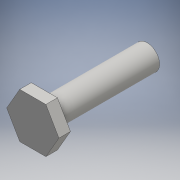
# Autodesk Inventor part: bolt
Saved by Autodesk Inventor 2016 (Build 200138000, 138)
## iProperties
Created: 2017-05-26
Part Number: bolt
Material: Ogólny
Document SubType Name: Modeling
Designer: Karol
Density: 1 g/cm^3
Appearance: Domyślna
Author: Karol
Autodesk Inventor part; units mm, degrees
ref_plane "YZ Plane" through (0, 0, 0) normal (1, 0, 0) x (0, 1, 0)
ref_plane "XZ Plane" through (0, 0, 0) normal (0, 1, 0) x (-1, 0, 0)
ref_plane "XY Plane" through (0, 0, 0) normal (0, 0, 1) x (1, 0, 0)
sketch "Sketch1" plane through (0, 0, 0) normal (0, 1, 0) x (-1, 0, 0)
  circle A0 centre (0, 0) radius 1.5
  dimension "d0" = 3
  constraints: 1 centre point, 1 coincident
  measures "d0" diameter of A0
extrude "Extrusion1" add sketch "Sketch1" along normal blind 12.5
sketch "Sketch2" plane through (0, 0, 0) normal (0, -1, 0) x (1, 0, 0)
  line L0 (3.1754, 0) -> (1.5877, -2.75)
  line L1 (1.5877, -2.75) -> (-1.5877, -2.75)
  line L2 (-1.5877, -2.75) -> (-3.1754, 0)
  line L3 (-3.1754, 0) -> (-1.5877, 2.75)
  line L4 (-1.5877, 2.75) -> (1.5877, 2.75)
  line L5 (1.5877, 2.75) -> (3.1754, 0)
  point P0 (0, 0)
  point P1 (0, 0)
  dimension "d6" = 5.5
  constraints: 12 end point, 13 other
  measures "d6" distance between parallel lines of L5 L2
extrude "Extrusion2" add sketch "Sketch2" along normal blind 1.4
body "Solid1"
